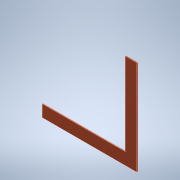
# Autodesk Inventor part: 8006_Cu_groundplane_Tx_Filter_Stage2_MPSv2_v1
Saved by Autodesk Inventor 2021 (Build 250183000, 183)
## iProperties
Created: 2021-04-07
Part Number: 8006_Cu_groundplane_Tx_Filter_Stage2_MPSv2_v1
Material: Copper
Document SubType Name: Modeling
Designer: Barksdale
Density: 8.94 g/cm^3
Appearance: Copper - Satin
Author: Barksdale
Autodesk Inventor part; units mm, degrees
ref_plane "YZ Plane" through (0, 0, 0) normal (1, 0, 0) x (0, 1, 0)
ref_plane "XZ Plane" through (0, 0, 0) normal (0, 1, 0) x (-1, 0, 0)
ref_plane "XY Plane" through (0, 0, 0) normal (0, 0, 1) x (1, 0, 0)
sketch "Sketch1" plane through (0, 0, 0) normal (0, 0, 1) x (1, 0, 0)
  line L0 (-17.8842, 30.4949) -> (102.1158, 30.4949)
  line L1 (102.1158, 30.4949) -> (102.1158, -89.5051)
  line L2 (102.1158, -89.5051) -> (-17.8842, -89.5051)
  line L3 (-17.8842, -89.5051) -> (-17.8842, 30.4949)
  line L4 (-17.8842, 30.4949) -> (87.1158, 30.4949)
  line L5 (87.1158, 30.4949) -> (87.1158, -74.5051)
  line L6 (87.1158, -74.5051) -> (-17.8842, -74.5051)
  line L7 (-17.8842, -74.5051) -> (-17.8842, 30.4949)
  point P0 (0, 0)
  point P1 (87.1158, 30.4949)
  point P2 (-17.8842, -74.5051)
  dimension "d0" = 120
  dimension "d1" = 120
  dimension "d2" = 105
  dimension "d3" = 105
  constraints: 16 end point, 4 parallel, 2 horizontal, 2 perpendicular
  measures "d0" distance of L1.end L2.end
  measures "d1" distance of L0.end L1.end
  measures "d2" distance of L5.end L6.end
  measures "d3" distance of L4.end L5.end
extrude "Extrusion1" add sketch "Sketch1" along normal blind 1 contours L0 L1 L2 L3 L6 L5
body "Solid1"
